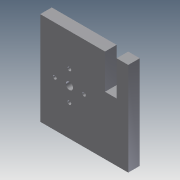
# Autodesk Inventor part: sidebasehole
Saved by Autodesk Inventor 2011 (Build 150239000, 239)
## iProperties
Created: 2011-12-10
Part Number: sidebasehole
Document SubType Name: Modeling
Designer: Matthew
Density: 1 g/cm^3
Author: Matthew
Autodesk Inventor part; units mm, degrees
ref_plane "YZ Plane" through (0, 0, 0) normal (1, 0, 0) x (0, 1, 0)
ref_plane "XZ Plane" through (0, 0, 0) normal (0, 1, 0) x (-1, 0, 0)
ref_plane "XY Plane" through (0, 0, 0) normal (0, 0, 1) x (1, 0, 0)
sketch "Sketch1" plane through (0, 0, 0) normal (0, 0, 1) x (1, 0, 0)
  line L0 (-21.2887, 16.8434) -> (23.7113, 16.8434)
  line L1 (23.7113, 16.8434) -> (23.7113, -34.1566)
  line L2 (23.7113, -34.1566) -> (-21.2887, -34.1566)
  line L3 (-21.2887, -34.1566) -> (-21.2887, 16.8434)
  point P0 (0, 0)
  dimension "d0" = 45
  dimension "d1" = 51
  constraints: 8 end point, 2 parallel, 1 horizontal, 1 perpendicular
  measures "d0" distance of L1.end L2.end
  measures "d1" distance of L0.end L1.end
extrude "Extrusion1" add sketch "Sketch1" along normal blind 3.175
sketch "Sketch2" plane through (0, 0, 3.175) normal (0, 0, 1) x (1, 0, 0)
  line L0 (-21.2887, -34.1566) -> (-21.2887, 16.8434) projected
  line L1 (-21.2887, -34.1566) -> (-21.2887, -9.1566)
  circle A0 centre (-5.2887, -9.1566) radius 8
  circle A1 centre (-13.2887, -9.1566) radius 1
  circle A2 centre (-5.2887, -1.1566) radius 1
  circle A3 centre (2.7113, -9.1566) radius 1
  circle A4 centre (-5.2887, -17.1566) radius 1
  point P0 (0, 0)
  dimension "d4" = 25
  dimension "d6" = 16
  dimension "d7" = 2
  dimension "d8" = 2
  dimension "d9" = 2
  dimension "d10" = 2
  dimension "d11" = 16
  constraints: 5 centre point, 4 point on circle, 2 end point, 1 point on line
  measures "d4" distance of L0.start L1.end
  measures "d6" diameter of A0
  measures "d7" diameter of A1
  measures "d8" diameter of A2
  measures "d9" diameter of A3
  measures "d10" diameter of A4
  measures "d11" distance of A0.centre L1.end
extrude "Extrusion2" cut sketch "Sketch2" against normal blind 25.4 contours A0 A3 | A0 A3 | A2 A0 | A0 A2 | A4 A0 | A0 A4 | A1 A0 | A0 A1
sketch "Sketch3" plane through (0, 0, 3.175) normal (0, 0, 1) x (1, 0, 0)
  circle A0 centre (-5.2887, -9.1566) radius 1.9812
  point P0 (0, 0)
  dimension "d14" = 3.9624
  constraints: 1 centre point
  measures "d14" diameter of A0
extrude "Extrusion3" cut sketch "Sketch3" against normal blind 25.4
sketch "Sketch4" plane through (0, 0, 0) normal (0, 0, -1) x (-1, 0, 0)
  circle A0 centre (5.2887, -9.1566) radius 1.9812 projected
  circle A1 centre (5.2887, -17.1566) radius 1 projected
  circle A2 centre (13.2887, -9.1566) radius 1 projected
  circle A3 centre (5.2887, -1.1566) radius 1 projected
  circle A4 centre (-2.7113, -9.1566) radius 1 projected
  line L0 (21.2887, 16.8434) -> (-23.7113, 16.8434) projected
  line L1 (-23.7113, 16.8434) -> (-23.7113, -34.1566) projected
  line L2 (-23.7113, -34.1566) -> (21.2887, -34.1566) projected
  line L3 (21.2887, -34.1566) -> (21.2887, 16.8434) projected
  line L4 (-23.7113, -34.1566) -> (-17.3613, -34.1566)
  point P0 (0, 0)
  dimension "d17" = 6.35
  constraints: 2 end point, 1 point on line
  measures "d17" distance of L1.end L4.end
extrude "Extrusion4" add sketch "Sketch4" along normal blind 3.175
sketch "Sketch5" plane through (23.7113, -34.1566, 3.175) normal (1, 0, 0) x (0, 0, -1)
  line L0 (0, 51) -> (0, 0) projected
  line L1 (0, 0) -> (6.35, 0) projected
  line L2 (6.35, 0) -> (6.35, 51) projected
  line L3 (0, 51) -> (6.35, 51) projected
  point P0 (3.175, 34.1566)
extrude "Extrusion5" add sketch "Sketch5" along normal blind 3.175
sketch "Sketch6" plane through (0, 0, 3.175) normal (0, 0, 1) x (1, 0, 0)
  line L0 (-21.2887, 16.8434) -> (26.8863, 16.8434) projected
  line L1 (26.8863, 16.8434) -> (20.5363, 16.8434)
  line L2 (20.5363, 16.8434) -> (14.1863, 16.8434)
  line L3 (14.1863, 16.8434) -> (14.1863, 4.1434)
  line L4 (14.1863, 4.1434) -> (20.5363, 4.1434)
  line L5 (20.5363, 4.1434) -> (20.5363, 16.8434)
  line L6 (14.1863, 4.1434) -> (20.5363, 4.1434)
  line L7 (20.5363, 4.1434) -> (20.5363, -2.2066)
  line L8 (20.5363, -2.2066) -> (14.1863, -2.2066)
  line L9 (14.1863, -2.2066) -> (14.1863, 4.1434)
  point P0 (0, 0)
  dimension "d22" = 6.35
  dimension "d23" = 6.35
  dimension "d24" = 12.7
  dimension "d25" = 6.35
  constraints: 18 end point, 4 parallel, 2 horizontal, 2 perpendicular, 1 point on line
  measures "d22" distance of L0.end L1.end
  measures "d23" distance of L4.end L3.end
  measures "d24" distance of L3.end L2.end
  measures "d25" distance of L6.end L7.end
extrude "Extrusion6" cut sketch "Sketch6" against normal blind 25.4
body "Solid1"
